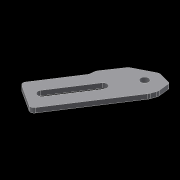
# Autodesk Inventor part: PelvisSubLinkLeft
Saved by Autodesk Inventor 2015 (Build 190159000, 159)
## iProperties
Created: 2014-12-04
Part Number: PelvisSubLinkLeft
Material: Generic
Document SubType Name: Modeling
Designer: Val
Density: 1 g/cm^3
Appearance: Default
Mass: 7.05234 g
Surface Area: 46.8232 cm^2
Volume: 7.05234 cm^3
Author: Val
Autodesk Inventor part; units mm, degrees
ref_plane "YZ Plane" through (0, 0, 0) normal (1, 0, 0) x (0, 1, 0)
ref_plane "XZ Plane" through (0, 0, 0) normal (0, 1, 0) x (-1, 0, 0)
ref_plane "XY Plane" through (0, 0, 0) normal (0, 0, 1) x (1, 0, 0)
sketch "Body" plane through (0, 0, 0) normal (0, 0, 1) x (1, 0, 0)
  line L0 (27.316, 36.0942) -> (2.7256, -1.7701) construction
  line L1 (-2.7256, 1.7701) -> (21.8647, 39.6345) construction
  line L2 (39.19, 35.3599) -> (32.4946, 58.4071) construction
  line L3 (32.4946, 58.4071) -> (19.5232, 59.2689) construction
  line L4 (19.5232, 59.2689) -> (15.4488, 53.2513) construction
  arc A0 (15.4488, 53.2513) -> (14.6202, 51.0054) centre (19.5891, 50.448) ccw
  line L5 (14.6202, 51.0054) -> (14.2763, 47.9393)
  arc A1 (13.5008, 45.7735) -> (14.2763, 47.9393) centre (9.3074, 48.4968) ccw
  line L6 (13.5008, 45.7735) -> (-11.4127, 7.4118) construction
  line L7 (11.4127, -7.4118) -> (39.19, 35.3599) construction
  line L8 (-11.4127, 7.4118) -> (11.4127, -7.4118) construction
  arc A2 (53.351, 57.1651) -> (54.2815, 59.0478) centre (45.8031, 62.067) ccw
  arc A3 (27.3464, 69.3874) -> (24.9347, 67.2614) centre (30.251, 63.6618) ccw
  arc A4 (45.1456, 77.1234) -> (42.0612, 76.8523) centre (43.9732, 72.7788) ccw
  arc A5 (54.9347, 73.4976) -> (53.8348, 74.7787) centre (53.444, 73.3305) ccw
  arc A6 (55.6234, 62.816) -> (55.882, 65.0506) centre (50.9132, 64.4933) ccw
  line L9 (42.0612, 76.8523) -> (27.3464, 69.3874)
  line L10 (53.8348, 74.7787) -> (45.1456, 77.1234)
  line L11 (55.882, 65.0506) -> (54.9347, 73.4976)
  line L12 (54.2815, 59.0478) -> (55.6234, 62.816)
  line L13 (39.19, 35.3599) -> (53.351, 57.1651)
  arc A7 (15.4488, 53.2513) -> (14.6202, 51.0054) centre (19.5891, 50.448) ccw
  line L14 (14.6202, 51.0054) -> (14.2763, 47.9393)
  line L15 (13.5008, 45.7735) -> (-3.2428, 19.9917)
  line L16 (-3.2428, 19.9917) -> (19.5825, 5.1682)
  line L17 (19.5825, 5.1682) -> (39.19, 35.3599)
  line L18 (24.9347, 67.2614) -> (15.4488, 53.2513)
  line L19 (27.316, 36.0942) -> (21.8647, 39.6345) construction
  circle A8 centre (13.6164, 20.9665) radius 3.25
  line L20 (13.6164, 20.9665) -> (34.175, 52.6228) construction
  circle A9 centre (28.7285, 44.2362) radius 3.25
  line L21 (26.0028, 46.0064) -> (10.8907, 22.7366)
  line L22 (31.4541, 42.4661) -> (16.342, 19.1964)
  circle A10 centre (42.1456, 66.1234) radius 3.25
  point P0 (0, 0)
  point P1 (0, 0)
  dimension "d25" = 138
  dimension "d26" = 111.5
  dimension "d27" = 154
  dimension "d31" = 6.5
  dimension "d32" = 15
  dimension "d33" = 16.5
  dimension "d34" = 151
  dimension "d35" = 6.4202
  dimension "d36" = 8.5
  dimension "d37" = 4
  dimension "d38" = 9
  dimension "d39" = 4.5
  dimension "d40" = 1.5
  dimension "d41" = 5
  dimension "d42" = 9
  dimension "d43" = 26
  dimension "d44" = 6.5
  dimension "d45" = 10
  dimension "d46" = 10
  dimension "d47" = 6.5
  dimension "d48" = 3
  dimension "d49" = 11
  constraints: 46 end point, 21 point on circle, 17 tangent, 13 centre point, 8 point on line, 4 parallel, 3 perpendicular, 2 collinear, 2 equal radius, 1 coincident, 1 midpoint, 9 other
  measures "d25" angle of L10 L9
  measures "d26" angle of L11 L10
  measures "d27" angle of L12 L11
  measures "d31" distance between parallel lines of L0 L1
  measures "d32" distance between parallel lines of L16 L8
  measures "d33" distance of L9.start L9.end
  measures "d34" angle of L9 L18
  measures "d35" radius of A3
  measures "d36" distance of L11.start L11.end
  measures "d37" distance of L12.start L12.end
  measures "d38" distance of L10.start L10.end
  measures "d39" radius of A4
  measures "d40" radius of A5
  measures "d41" radius of A6
  measures "d42" radius of A2
  measures "d43" distance of L2.start L13.end
  measures "d44" diameter of A8
  measures "d45" distance from line of L16 L20.start
  measures "d46" distance of A9.centre L20.end
  measures "d47" diameter of A10
  measures "d48" horizontal distance of A10.centre L10.end
  measures "d49" vertical distance of A10.centre L10.end
extrude "BodyFeature" add sketch "Body" along normal blind 4
fillet "EndFilletsFeature" radius 3 2 edges at (-3.2428, 19.9917, 2) (19.5825, 5.1682, 2)
